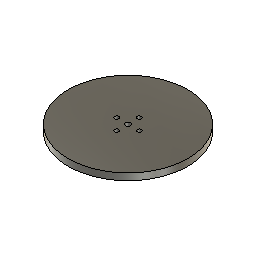
115mm-wheel (Autodesk Fusion 360 design; units mm, degrees)
Autodesk Fusion 360 part; units mm, degrees
sketch "Sketch1" plane through (0, 0, 0) normal (0, 0, 1) x (1, 0, 0)
  circle A0 centre (0, 0) radius 57.5
  circle A1 centre (0, 0) radius 2.5
  line L0 (0, 0) -> (0, 10.87) construction
  circle A2 centre (0, 10.87) radius 2
  circle A3 centre (-10.87, 0) radius 2
  circle A4 centre (0, -10.87) radius 2
  circle A5 centre (10.87, 0) radius 2
  dimension "d1" = 115
  dimension "d2" = 5
  dimension "d3" = 10.87
  dimension "d4" = 4
  dimension "d6" = 360
  constraint coincident A0.centre A1.centre
  constraint vertical L0
  constraint coincident L0.end A2.centre
  measures "d1" diameter of A0
  measures "d2" diameter of A1
  measures "d3" distance of A0.centre L0.end
  measures "d4" diameter of A2
extrude "Extrude1" add sketch "Sketch1" along normal blind 6.5
